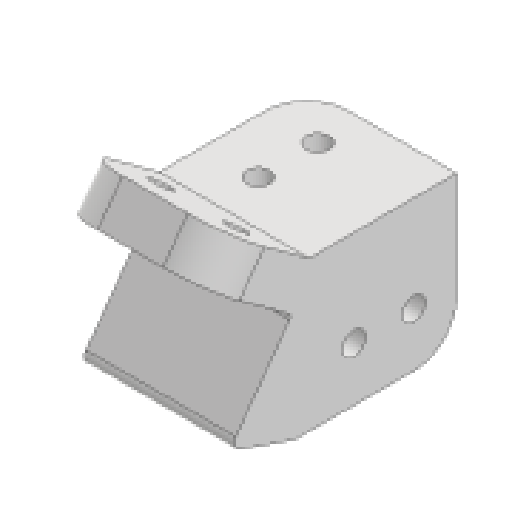
# Autodesk Inventor part: upperRearBracket
Saved by Autodesk Inventor 2025 (Build 290162000, 162)
## iProperties
Created: 2024-12-14
Part Number: upperRearBracket
Material: Generic
Document SubType Name: Modeling
Designer: derm
Density: 1 g/cm^3
Appearance: Default
Author: derm
Autodesk Inventor part; units mm, degrees
ref_plane "YZ Plane" through (0, 0, 0) normal (1, 0, 0) x (0, 1, 0)
ref_plane "XZ Plane" through (0, 0, 0) normal (0, 1, 0) x (-1, 0, 0)
ref_plane "XY Plane" through (0, 0, 0) normal (0, 0, 1) x (1, 0, 0)
sketch "Sketch1" plane through (0, 0, 0) normal (1, 0, 0) x (0, 1, 0)
  line L0 (0, 0) -> (25.4, 0)
  line L1 (25.4, 0) -> (25.4, -38.1)
  line L2 (25.4, -38.1) -> (0, -38.1)
  line L3 (0, -38.1) -> (0, 0)
  circle A0 centre (12.7, -27.9675) radius 2.75
  circle A1 centre (12.7, -13.8886) radius 2.75
  dimension "d0" = 25.4
  dimension "d1" = 38.1
  dimension "d2" = 5.5
  constraints: 8 end point, 2 centre point, 2 parallel, 1 equal radius, 1 horizontal, 1 perpendicular
  measures "d0" distance of L0.start L0.end
  measures "d1" distance of L0.end L1.end
  measures "d2" diameter of A0
extrude "Extrusion1" add sketch "Sketch1" along normal blind 10
sketch "Sketch2" plane through (10, 0, 0) normal (1, 0, 0) x (0, 0, -1)
  line L0 (-11.9576, 10.5414) -> (-13.9859, 7.7441) projected
  line L1 (-2.4758, 23.6177) -> (-4.5041, 20.8204) projected
  line L2 (-18.0308, 7.0996) -> (-20.828, 9.1279) projected
  line L3 (-31.1071, 16.5813) -> (-33.9043, 18.6096) projected
  line L4 (-34.5489, 22.6546) -> (-32.5206, 25.4518) projected
  line L5 (-25.0672, 35.7309) -> (-23.0389, 38.5281) projected
  line L6 (-3.1204, 27.6626) -> (-5.9176, 29.6909) projected
  line L7 (-16.1967, 37.1443) -> (-18.9939, 39.1726) projected
  line L8 (38.1, 0) -> (38.1, 25.4) projected
  line L9 (38.1, 25.4) -> (0, 25.4) projected
  line L10 (0, 25.4) -> (0, 0) projected
  line L11 (0, 0) -> (38.1, 0) projected
  circle A0 centre (13.8886, 12.7) radius 2.75 projected
  circle A1 centre (27.9675, 12.7) radius 2.75 projected
  line L12 (-0.7756, 25.9624) -> (-21.3387, 40.8728)
  line L13 (-0.7756, 25.9624) -> (0, 25.4)
  line L14 (-15.6861, 5.3994) -> (-0.7756, 25.9624)
  line L15 (-15.6861, 5.3994) -> (0, 0)
  line L16 (-15.6861, 5.3994) -> (-36.2491, 20.3098)
  line L17 (-21.3387, 40.8728) -> (-15.4684, 48.9685)
  line L18 (-15.4684, 48.9685) -> (17.7637, 24.8716)
  line L19 (17.7637, 24.8716) -> (11.8935, 16.7759)
  line L20 (11.8935, 16.7759) -> (-21.3387, 40.8728)
  line L21 (-15.6861, 5.3994) -> (-36.2491, 20.3098)
  line L22 (38.1, 0) -> (0, 0)
  line L23 (38.1, 25.4) -> (38.1, 35.4)
  line L24 (38.1, 35.4) -> (1.1477, 35.4)
  line L25 (1.1477, 35.4) -> (1.1477, 25.4)
  line L26 (1.1477, 25.4) -> (38.1, 25.4)
  point P0 (17.035, 25.4)
  point P1 (3.244, 35.4)
  dimension "d5" = 10
  dimension "d10" = 10
  constraints: 30 end point, 5 equal length, 4 perpendicular
  measures "d5" distance of L12.end L17.end
  measures "d10" distance between parallel lines of L24 L9
extrude "Extrusion2" add sketch "Sketch2" against normal blind 35.4 contours L14 L1 L13 L10 L15 L0 | L12 L6 L7 L17 L18 L24 L25 L9 L13 | L25 L24 L18 L9 | L9 L18 L24 L23
sketch "Sketch3" plane through (0, 25.4, -38.1) normal (0, -1, 0) x (1, 0, 0)
  line L0 (0, 0) -> (0, 38.1) projected
  line L1 (0, 38.1) -> (-25.4, 38.1) projected
  line L2 (-25.4, 0) -> (-25.4, 38.1) projected
  line L3 (0, 0) -> (-25.4, 0) projected
  line L4 (10, 12.8825) -> (10, 7.3825) projected
  line L5 (0, 12.8825) -> (0, 7.3825) projected
  line L6 (10, 26.9614) -> (10, 21.4614) projected
  circle A0 centre (-12.7, 10.1325) radius 2.75
  circle A1 centre (-12.7, 24.2114) radius 2.75
  point P0 (0, 38.1)
  constraints: 2 centre point
extrude "Extrusion3" cut sketch "Sketch3" against normal blind 35.4 contours A0 | A1
sketch "Sketch4" plane through (-25.4, 40.8728, 21.3387) normal (0, -0.8096, 0.587) x (1, 0, 0)
  line L0 (35.4, 0) -> (35.4, -25.4) projected
  line L1 (35.4, 0) -> (0, 0) projected
  line L2 (0, -25.4) -> (0, 0) projected
  line L3 (35.4, -25.4) -> (0, -25.4) projected
  line L4 (26.667, -12.7) -> (8.9084, -12.7) construction
  line L5 (26.667, -10.1) -> (8.9084, -10.1)
  line L6 (8.9084, -15.3) -> (26.667, -15.3)
  arc A0 (26.667, -15.3) -> (26.667, -10.1) centre (26.667, -12.7) ccw
  arc A1 (8.9084, -10.1) -> (8.9084, -15.3) centre (8.9084, -12.7) ccw
  circle A2 centre (26.667, -12.7) radius 2.6
  circle A3 centre (8.9084, -12.7) radius 2.6
  point P0 (25.4, -41.2685)
  point P1 (17.7877, -12.7)
  point P2 (8.9084, -10.1)
  point P3 (26.667, -10.1)
  dimension "d13" = 2.6
  constraints: 8 end point, 4 point on circle, 4 tangent, 2 centre point, 2 coincident, 1 horizontal, 1 midpoint, 1 parallel, 6 other
  measures "d13" radius of A1
extrude "Extrusion4" cut sketch "Sketch4" against normal blind 35.4 contours A0 A2 | A3 A1
fillet "Fillet1" radius 10 4 edges at (5, 0, -38.1) (-25.4, 30.4, -38.1) (10, 44.9207, 18.4035) (-25.4, 44.9207, 18.4035)
fillet "Fillet2" radius 2 2 edges at (-12.7, 0, 0) (-7.7, 5.3994, 15.6861)
fillet "Fillet3" radius 1 1 edges at (-7.7, 25.9624, 0.7756)
body "Solid1"
